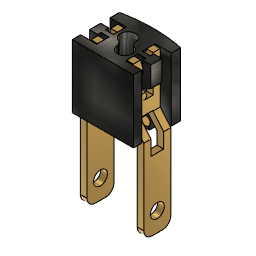
120v Plug (Autodesk Fusion 360 design; units mm, degrees)
Autodesk Fusion 360 part; units mm, degrees
sketch "Base Outline" plane through (0, 0, 0) normal (0, 0, 1) x (1, 0, 0)
  line L0 (-7.5, 25.5) -> (-5.5, 25.5)
  line L1 (-6, 32) -> (-7.5, 32)
  line L2 (6, 26) -> (7.5, 26)
  line L3 (-5.5, 32.5) -> (-7.5, 32.5)
  line L4 (6, 32) -> (6, 26)
  line L5 (7.5, 32.5) -> (5.5, 32.5)
  line L6 (7.5, 26) -> (7.5, 32)
  line L7 (-7.5, 26) -> (-6, 26)
  line L8 (-7.5, 32) -> (-7.5, 26)
  line L9 (5.5, 25.5) -> (7.5, 25.5)
  line L10 (-5.5, 25.5) -> (-5.5, 32.5)
  line L11 (7.5, 32) -> (6, 32)
  line L12 (-10.5, 33.9116) -> (-10.5, 20.3453)
  circle A0 centre (0, 0) radius 38
  line L13 (10.5, 20.3453) -> (10.5, 33.9116)
  line L14 (-7.5, 34.6987) -> (-7.5, 23.3453)
  circle A1 centre (0, 0) radius 35.5
  line L15 (-6, 26) -> (-6, 32)
  line L16 (5.5, 32.5) -> (5.5, 25.5)
  line L17 (-10.5, 20.3453) -> (10.5, 20.3453)
  line L18 (-7.5, 23.3453) -> (7.5, 23.3453)
  line L19 (7.5, 23.3453) -> (7.5, 34.6987)
  line L20 (-7.25, 34.7518) -> (-7.25, 23.5953)
  line L21 (-7.25, 23.5953) -> (7.25, 23.5953)
  line L22 (7.25, 23.5953) -> (7.25, 34.7518)
  dimension "d1" = 0.5
  dimension "d2" = 0.5
  constraint coincident L12.start A1
  constraint coincident L14.start A1
  constraint coincident L14.end L18
  constraint coincident L18.start L14
  constraint coincident L13.end A1
  constraint coincident L19.end A1
  constraint collinear L8 L14
  constraint collinear L6 L19
  constraint parallel L5 L11
  constraint parallel L4 L16
  constraint parallel L2 L9
  constraint coincident L19 L9.end
  constraint coincident L19 L5.start
  constraint parallel L0 L7
  constraint parallel L10 L15
  constraint parallel L1 L3
  constraint coincident L14 L0.start
  constraint coincident L14 L3.end
  constraint parallel L14 L20
  constraint parallel L18 L21
  constraint parallel L19 L22
  constraint coincident A1 L22.end
  constraint coincident A1 L20.start
extrude "Extrude1" add sketch "Base Outline" along normal blind 15 contours L0 L1 L3 L7 L10 L15 L20 | L0 L3 L5 L9 L10 A1 L16 L20 L21 L22 | L1 L7 L15 L20 | L2 L4 L5 L9 L11 L16 L22 | L2 L4 L11 L22 makes body 1 in component "Plug Housing"
sketch "Sketch1" plane through (0, 0, 0) normal (0, 1, 0) x (1, 0, 0) in component "Leads"
  line L0 (0, 20) -> (0, -15) construction
  line L1 (-7.5, -15) -> (7.5, -15) construction
  line L2 (7.5, -15) -> (7.5, -3)
  line L3 (10, 20) -> (10, 0)
  line L4 (0, 20) -> (17.0294, 20) construction
  line L5 (10, 0) -> (7.5, -3)
  line L6 (8.43, 20) -> (8.43, 0.5684)
  line L7 (8.43, 0.5684) -> (5.93, -2.4316)
  line L8 (5.93, -15) -> (5.93, -2.4316)
  line L9 (8.43, 20) -> (10, 20)
  line L10 (5.93, -15) -> (10, -15)
  line L11 (10, 0) -> (10, -15)
  dimension "d6" = 35
  dimension "d7" = 12
  dimension "d8" = 18.8
  dimension "d9" = 3
  dimension "d10" = 2.5
  dimension "d11" = 1.57
  constraint vertical L0
  constraint coincident L0.end L1
  constraint midpoint L0.end L1
  constraint coincident L1.end L2.start
  constraint perpendicular L1 L2
  constraint parallel L0 L3
  constraint horizontal L4
  constraint coincident L3.start L4
  constraint perpendicular L3 L9
  constraint perpendicular L2 L10
  constraint parallel L3 L11
  measures "d6" distance of L0.end L0.start
  measures "d7" distance of L1.end L2.end
  measures "d9" vertical distance of L2.end L3.end
  measures "d10" distance of L2 L3
extrude "Extrude1'" add sketch "Sketch1" along normal blind 6.4 separate body contours L2 L3 L5 L6 L7 L8 L9 L10 makes body 2 in component "Leads"
fillet "Fillet1" radius 2 2 edges at (9.215, 0, -20) (9.215, 6.4, -20) on bodies 2 in component "Leads"
sketch "Sketch2" plane through (10, 0, 0) normal (1, 0, 0) x (0, 1, 0) in component "Leads"
  arc A0 (4.4, -20) -> (6.4, -18) centre (4.4, -18) ccw
  line L0 (6.4, -18) -> (6.4, 0)
  line L1 (6.4, 0) -> (0, 0)
  line L2 (0, 0) -> (0, -18)
  arc A1 (0, -18) -> (2, -20) centre (2, -18) ccw
  line L3 (2, -20) -> (4.4, -20)
  arc A2 (4.4, -20) -> (6.4, -18) centre (4.4, -18) ccw
  line L4 (2, -20) -> (4.4, -20)
  arc A3 (0, -18) -> (2, -20) centre (2, -18) ccw
  line L5 (0, 15) -> (6.4, 15)
  line L6 (0, 15) -> (0, 2.4316)
  line L7 (6.4, 2.4316) -> (6.4, 15)
  line L8 (0, -0.5684) -> (0, 2.4316)
  line L9 (6.4, -0.5684) -> (6.4, 2.4316)
  line L10 (0, -18) -> (0, -0.5684)
  line L11 (6.4, -18) -> (6.4, -0.5684)
  line L12 (3.2, 15) -> (3.2, -20) construction
  line L13 (1.7015, 15) -> (1.7015, 6.3)
  line L14 (0, 6.3) -> (6.4, 6.3)
  line L15 (4.6985, 15) -> (4.6985, 6.3)
  line L16 (0, 12.6) -> (2.4, 12.6)
  line L17 (2.4, 12.6) -> (1.7015, 15)
  line L18 (4, 12.6) -> (4.6985, 15)
  line L19 (4, 12.6) -> (6.4, 12.6)
  circle A4 centre (2.4445, 7.0415) radius 0.75
  circle A5 centre (2.4672, 2.3667) radius 0.75
  line L20 (6.4, 3.15) -> (0, 3.15)
  line L21 (1.7015, 6.3) -> (1.7015, -3.55)
  line L22 (4.6985, 6.3) -> (4.6985, -3.55)
  line L23 (0, -3.55) -> (6.4, -3.55)
  circle A6 centre (3.2, -15.4) radius 1.65
  line L24 (2.6903, 12.2784) -> (2.6903, 15)
  line L25 (2.6903, 15) -> (3.7097, 15)
  line L26 (3.7097, 15) -> (3.7097, 12.2784)
  line L27 (3.2, 13.6111) -> (2.6903, 15) construction
  line L28 (3.2, 13.6111) -> (3.7097, 15) construction
  line L29 (4.5095, 12.2784) -> (4.5095, 8.1307)
  line L30 (4.5095, 8.1307) -> (1.8905, 8.1307)
  line L31 (1.8905, 8.1307) -> (1.8905, 12.2784)
  line L32 (1.8905, 12.2784) -> (2.6903, 12.2784)
  line L33 (3.7097, 12.2784) -> (4.5095, 12.2784)
  point P0 (2.557, 6.3)
  dimension "d15" = 8.7
  dimension "d16" = 2.4
  dimension "d17" = 2.4
  dimension "d18" = 1.5
  dimension "d19" = 1.5
  dimension "d21" = 3.3
  dimension "d22" = 4.6
  constraint midpoint L5 L12.start
  constraint midpoint L4 L12.end
  constraint coincident L5 L13.start
  constraint perpendicular L1 L13
  constraint perpendicular L7 L14
  constraint coincident L7 L14.end
  constraint coincident L6 L14.start
  constraint symmetric L12 L13.start L15.start
  constraint symmetric L12 L13.end L15.end
  constraint coincident L6 L16.start
  constraint perpendicular L13 L16
  constraint symmetric L12 L16.end L18.start
  constraint perpendicular L7 L19
  constraint coincident L7 L19.end
  constraint coincident A4 P0
  constraint coincident L14 P0
  constraint coincident L6 L20.end
  constraint perpendicular L6 L20
  constraint perpendicular L1 L21
  constraint perpendicular L1 L22
  constraint perpendicular L0 L23
  constraint coincident L0 L23.end
  constraint coincident L2 L23.start
  constraint coincident L12 A6.centre
  constraint parallel L24 L26
  constraint coincident L12 L27.start
  constraint collinear L5 L25
  constraint horizontal L32
  constraint vertical L29
  constraint horizontal L30
  constraint vertical L31
  constraint symmetric L12 L29 L31
  constraint collinear L32 L33
  measures "d15" distance of L13.start L13.end
  measures "d16" distance of L16.start L16.end
  measures "d17" distance of L13.start L16
  measures "d18" diameter of A4
  measures "d19" diameter of A5
  measures "d21" diameter of A6
  measures "d22" distance of L4 A6.centre
extrude "Extrude2" cut sketch "Sketch2" against normal blind 15 contours L1 L21 L22 L23 | L1 L20 L21 L22 | L5 L13 L14 L15 L16 L17 L18 L19 A4 L24 L26 L29 L30 L31 L32 L33 | L5 L24 L25 L26 L29 L30 L31 L32 L33 | A6 bodies 2 makes body 3 at (7.0987, 3.0993, 2.7704) in component "Leads"
extrude "Extrude3" add sketch "Sketch2" against normal blind 4.7 from surface at -4.07 contours L14 A4 | L13 L14 A4 | L13 A4 | A5 picked at (2.1815, 7.4062) bodies 3 2 in component "Leads"
chamfer "Chamfer1" distance 0.6 distance2 4.1 2 edges at (1.23, 1.7452, 7.3127) (1.23, 1.7679, 2.6379) measured on face at (1.23, 2.384, 7.2532) measured on face at (1.23, 2.5811, 2.564) on bodies 2 3 in component "Leads"
copy_body "Body->Comp1" bodies 2 removing the originals makes body 4 in component "Right"
extrude "Extrude2'" cut sketch "Sketch1" along normal blind 7 from surface at -0.25 sketch seen with x (1, 0, 0) y (0, 1, 0) z (0, 0, 1) at (-2.5, 25.8, 0) bodies 1 in component "Plug Housing"
extrude "Extrude3'" add sketch "Sketch2" against normal up to surface (3.82 mm away) from surface at -0.25 contours L5 L24 L25 L26 L29 L30 L31 L32 L33 sketch seen with x (1, 0, 0) y (0, 1, 0) z (0, 0, 1) at (-2.5, 25.8, 0) bodies 1 in component "Plug Housing"
mirror "Mirror1" about plane through (0, 0, 0) normal (1, 0, 0) of 12 faces at (4.7809, 30.2167, 0.8105) (5.9767, 25.55, 5.8105) (3.43, 29.4698, 4.3313) (5.9767, 32.55, 5.8105) (5.9767, 30.3095, 10.8958) (4.7033, 30.0429, 12.2784) (5.9767, 29.5097, 14.0928) (7.25, 29.1699, 9.5133) (5.9767, 28.4903, 13.1856) (4.7033, 28.2237, 12.2784) (5.9767, 27.6905, 9.5133) (5.9767, 29.4365, 8.1307) on bodies 1 in component "Plug Housing"
sketch "Sketch3" plane through (0, 0, 0) normal (0, 0, 1) x (1, 0, 0) in component "Leads"
  line L0 (-5, -2.4547) -> (10, -2.4547)
  line L1 (10, -2.4547) -> (10, 8.8987)
  line L2 (-5, 8.8987) -> (-5, -2.4547)
  circle A0 centre (1.4374, 4.7655) radius 1.75
  circle A1 centre (3.545, 1.9713) radius 1.75
  line L3 (-0.93, 6.75) -> (-4.75, 6.75)
  line L4 (5.93, 6.75) -> (9.75, 6.75)
  line L5 (5.93, 0) -> (5.93, 6.75)
  line L6 (-0.93, 6.75) -> (-0.93, 0)
  line L7 (-0.93, 3.375) -> (5.93, 3.375) construction
  line L8 (10, 0) -> (-5, 0)
  line L9 (3.545, 1.9713) -> (1.4374, 4.7655) construction
  line L10 (1.801, 2.1155) -> (1.0969, 3.0489)
  line L11 (3.8855, 3.6878) -> (3.1814, 4.6213)
  point P0 (10, 0)
  point P1 (2.5, 6.625)
  point P2 (2.5, 0.125)
  point P3 (2.5, 3.375)
  point P4 (2.5, 3.375)
  dimension "d39" = 3.5
  dimension "d40" = 3.5
  dimension "d58" = 3.4999
  constraint coincident L4.start L5.end
  constraint coincident L3.start L6.start
  constraint coincident L5 L7.end
  constraint coincident P0 L8.start
  constraint coincident L2 L8.end
  constraint perpendicular L2 L8
  constraint coincident L8 L5.start
  constraint coincident L6 L7.start
  constraint coincident L8 L6.end
  constraint vertical L5
  constraint horizontal L7
  constraint midpoint L5 L7.end
  constraint coincident A0 P4
  constraint coincident A1 P4
  constraint coincident P4 P3
  constraint coincident L7 P4
  constraint midpoint L7 P4
  constraint coincident A1.centre L9.start
  constraint coincident A0.centre L9.end
  constraint coincident A1 L10.start
  constraint coincident A0 L10.end
  constraint parallel L9 L10
  constraint symmetric L9 L10.start L11.start
  constraint symmetric L9 L10.end L11.end
  measures "d39" diameter of A0
  measures "d40" diameter of A1
  measures "d58" distance of A1.centre A0.centre
extrude "Extrude5" cut sketch "Sketch3" against normal blind 13 from surface at 15 contours A0 | A0 A1 L10 | A0 A1 L11 | A1 sketch seen with x (1, 0, 0) y (0, 1, 0) z (0, 0, 1) at (-2.5, 25.8, 0) bodies 1 in component "Plug Housing"
sketch "Sketch2 (2)" plane through (0, 0, 0) normal (0, 0, 1) x (1, 0, 0)
  line L0 (-7.25, 27.6905) -> (-5.4563, 27.6905)
  line L1 (-7.25, 27.6905) -> (-7.25, 30.3095)
  line L2 (-7.25, 30.3095) -> (-5.4563, 30.3095)
  line L3 (-7.25, 32.55) -> (-5.4563, 32.55)
  line L4 (-5.4563, 32.55) -> (-5.4563, 30.3095)
  line L5 (-5.4563, 27.6905) -> (-5.4563, 25.55)
  line L6 (-5.4563, 25.55) -> (-7.25, 25.55)
  line L7 (-7.25, 34.7518) -> (-7.25, 32.55)
  arc A0 (7.25, 34.7518) -> (-7.25, 34.7518) centre (0, 0) ccw
  line L8 (7.25, 32.55) -> (7.25, 34.7518)
  line L9 (7.25, 32.55) -> (5.4563, 32.55)
  line L10 (5.4563, 32.55) -> (5.4563, 30.3095)
  line L11 (5.4563, 27.6905) -> (5.4563, 25.55)
  line L12 (5.4563, 25.55) -> (7.25, 25.55)
  line L13 (7.25, 23.5953) -> (7.25, 25.55)
  line L14 (-7.25, 23.5953) -> (7.25, 23.5953)
  line L15 (-7.25, 25.55) -> (-7.25, 23.5953)
  line L16 (7.25, 27.6905) -> (5.4563, 27.6905)
  line L17 (7.25, 30.3095) -> (5.4563, 30.3095)
  line L18 (7.25, 30.3095) -> (7.25, 27.6905)
  line L19 (5.4946, 27.35) -> (1.1188, 27.35)
  line L20 (1.1188, 27.35) -> (1.1188, 29.15)
  line L21 (5.4563, 32.55) -> (5.4563, 25.55)
  line L22 (1.1188, 29.15) -> (5.4563, 29.15)
  line L23 (-7.25, 29) -> (7.25, 29) construction
  line L24 (0, 23.5953) -> (0, 35.5) construction
  line L25 (-5.4563, 30.75) -> (-1.1188, 30.75)
  line L26 (-1.1188, 30.75) -> (-1.1188, 28.95)
  line L27 (-1.1188, 28.95) -> (-5.4563, 28.95)
  line L28 (-5.4563, 28.95) -> (-5.4563, 30.75)
  line L29 (-7.25, 32.55) -> (0.5, 32.55)
  dimension "d47" = 1.8
  dimension "d49" = 1.8
  dimension "d52" = 1.8
  constraint perpendicular L11 L19
  constraint perpendicular L19 L20
  constraint coincident L21 L22.end
  constraint perpendicular L21 L22
  constraint midpoint L1 L23.start
  constraint perpendicular L18 L23
  constraint coincident L18 L23.end
  constraint midpoint L14 L24.start
  constraint perpendicular L14 L24
  constraint coincident A0 L24.end
  constraint coincident L4 L25.start
  constraint perpendicular L25 L28
  constraint coincident L3.start L7.end
  constraint perpendicular L24 L29
  measures "d47" distance of L12 L19
  measures "d49" distance of L19 L22
  measures "d52" distance of L25 L29
extrude "Extrude6" cut sketch "Sketch2 (2)" along normal blind 8 contours L4 L25 L26 L27 L28 | L11 L19 L20 L21 L22 bodies 1 in component "Plug Housing"
chamfer "Chamfer1'" distance 3.8 distance2 2 2 edges at (7.25, 29, 8.1307) (-7.25, 29, 8.1307) measured on face at (5.9767, 29.4365, 8.1307) measured on face at (-5.9767, 29.4365, 8.1307) on bodies 1 in component "Plug Housing"
sketch "Sketch3 (2)" plane through (0, 0, 12.2784) normal (0, 0, 1) x (-1, 0, 0)
  line L0 (-3.43, -28.4903) -> (-3.43, -27.6905)
  line L1 (-3.43, -27.6905) -> (-7.25, -27.6905)
  line L2 (-7.25, -27.6905) -> (-7.25, -28.4903)
  line L3 (-7.25, -28.4903) -> (-3.43, -28.4903)
  line L4 (-7.25, -27.6905) -> (-3.43, -27.6905)
  line L5 (-7.25, -27.6905) -> (-7.25, -28.4903)
  line L6 (-7.25, -28.4903) -> (-3.43, -28.4903)
  line L7 (-7.25, -30.3095) -> (-3.43, -30.3095)
  line L8 (-7.25, -29.5097) -> (-7.25, -30.3095)
  line L9 (-7.25, -29.5097) -> (-3.43, -29.5097)
  line L10 (7.25, -27.6905) -> (3.43, -27.6905)
  line L11 (3.43, -32.55) -> (3.43, -25.8)
  line L12 (7.25, -28.4903) -> (7.25, -27.6905)
  line L13 (3.43, -28.4903) -> (7.25, -28.4903)
  line L14 (7.25, -30.3095) -> (3.43, -30.3095)
  line L15 (7.25, -30.3095) -> (7.25, -29.5097)
  line L16 (3.43, -29.5097) -> (3.43, -32.55)
  line L17 (-5.34, -30.3095) -> (-5.34, -29.5097)
  line L18 (-5.34, -28.4903) -> (-5.34, -27.6905)
  constraint midpoint L7 L17.start
  constraint midpoint L9 L17.end
  constraint midpoint L6 L18.start
  constraint midpoint L4 L18.end
extrude "Extrude7" add sketch "Sketch3 (2)" along normal up to surface (2.7216 mm away) contours L1 L2 L3 L4 L5 L6 L18 | L7 L8 L9 L17 bodies 1 in component "Plug Housing"
mirror "Mirror2" about plane through (0, 0, 0) normal (1, 0, 0) of "Extrude7" in component "Plug Housing"
component "Plug Housing" placed x (1, 0, 0) y (0, 1, 0) z (0, 0, 1) at (0, 0, 0)
component "Leads" placed x (1, 0, 0) y (0, 1, 0) z (0, 0, 1) at (-2.5, 25.8, 0)
component "Right" placed x (1, 0, 0) y (0, 1, 0) z (0, 0, 1) at (0, 0, 0) in component "Leads"
component "Right" placed x (-1, 0, 0) y (0, -1, 0) z (0, 0, 1) at (4.9912, 6.3575, 0) in component "Leads"
equation "d40 = d39"
